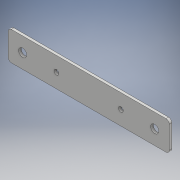
# Autodesk Inventor part: ramie1a
Saved by Autodesk Inventor 2017.3 (Build 213256000, 256)
## iProperties
Created: 2019-03-17
Part Number: ramie1a
Material: Ogólny
Document SubType Name: Modeling
Designer: legox
Density: 1 g/cm^3
Appearance: Domyślna
Author: legox
Autodesk Inventor part; units mm, degrees
ref_plane "YZ Plane" through (0, 0, 0) normal (1, 0, 0) x (0, 1, 0)
ref_plane "XZ Plane" through (0, 0, 0) normal (0, 1, 0) x (-1, 0, 0)
ref_plane "XY Plane" through (0, 0, 0) normal (0, 0, 1) x (1, 0, 0)
sketch "Szkic1" plane through (0, 0, 0) normal (0, 1, 0) x (-1, 0, 0)
  line L0 (-2, 0) -> (-98, 0)
  line L1 (-100, 2) -> (-100, 16)
  line L2 (-98, 18) -> (-2, 18)
  line L3 (0, 16) -> (0, 2)
  circle A0 centre (-9, 9) radius 2.5
  circle A1 centre (-30, 9) radius 1.5
  circle A2 centre (-91, 9) radius 2.5
  circle A3 centre (-70, 9) radius 1.5
  arc A4 (-2, 0) -> (0, 2) centre (-2, 2) ccw
  arc A5 (0, 16) -> (-2, 18) centre (-2, 16) ccw
  arc A6 (-100, 2) -> (-98, 0) centre (-98, 2) ccw
  arc A7 (-98, 18) -> (-100, 16) centre (-98, 16) ccw
  point P0 (0, 0)
  point P1 (-100, 18)
  point P2 (-100, 0)
  point P3 (0, 18)
  dimension "d0" = 100
  dimension "d1" = 18
  dimension "d2" = 5
  dimension "d3" = 9
  dimension "d4" = 9
  dimension "d5" = 3
  dimension "d6" = 9
  dimension "d7" = 30
  dimension "d8" = 2
  constraints: 8 centre point, 8 end point, 8 point on circle, 8 point on line, 8 tangent, 3 equal radius, 2 parallel, 1 horizontal, 1 perpendicular
  measures "d0" distance of point (-100, 18) point (0, 18)
  measures "d1" distance of point (-100, 0) point (-100, 18)
  measures "d2" diameter of A0
  measures "d3" distance from line of L3 A0.centre
  measures "d4" distance from line of L2 A0.centre
  measures "d5" diameter of A1
  measures "d6" distance from line of L2 A1.centre
  measures "d7" distance from line of L3 A1.centre
  measures "d8" radius of A4
extrude "Wyciągnięcie proste1" add sketch "Szkic1" along normal blind 1.6
equation "\"d4\" = 0.5 * d1"
equation "\"d6\" = d4"
